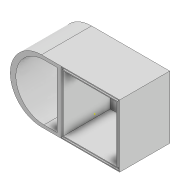
# Autodesk Inventor part: BetterPrototyp
Saved by Autodesk Inventor 2020 (Build 240168000, 168)
## iProperties
Created: 2021-06-29
Part Number: BetterPrototyp
Material: Generisch
Document SubType Name: Modeling
Designer: Julian Uhl
Density: 1 g/cm^3
Appearance: Vorgabe
Author: Julian Uhl
Autodesk Inventor part; units mm, degrees
ref_plane "YZ Plane" through (0, 0, 0) normal (1, 0, 0) x (0, 1, 0)
ref_plane "XZ Plane" through (0, 0, 0) normal (0, 1, 0) x (-1, 0, 0)
ref_plane "XY Plane" through (0, 0, 0) normal (0, 0, 1) x (1, 0, 0)
sketch "Skizze1" plane through (0, 0, 0) normal (0, 0, 1) x (1, 0, 0)
  line L0 (-160.1182, 0) -> (119.8818, 0) projected
  line L1 (0, -160.7697) -> (0, 119.2303) projected
  line L2 (-120.1182, 79.2303) -> (79.8818, 79.2303)
  line L3 (79.8818, 79.2303) -> (79.8818, -120.7697)
  line L4 (79.8818, -120.7697) -> (-120.1182, -120.7697)
  line L5 (-120.1182, -120.7697) -> (-120.1182, 79.2303)
  line L6 (-110.1182, 69.2303) -> (69.8818, 69.2303)
  line L7 (69.8818, 69.2303) -> (69.8818, -110.7697)
  line L8 (69.8818, -110.7697) -> (-110.1182, -110.7697)
  line L9 (-110.1182, -110.7697) -> (-110.1182, 69.2303)
  point P0 (0, 0)
  dimension "d0" = 200
  dimension "d1" = 200
  dimension "d2" = 10
  dimension "d3" = 10
  dimension "d4" = 10
  dimension "d5" = 10
  constraints: 16 end point, 4 parallel, 2 horizontal, 2 perpendicular
  measures "d0" distance between parallel lines of L4 L2
  measures "d1" distance between parallel lines of L5 L3
  measures "d2" distance between parallel lines of L2 L6
  measures "d3" distance between parallel lines of L5 L9
  measures "d4" distance between parallel lines of L3 L7
  measures "d5" distance between parallel lines of L4 L8
extrude "Extrusion1" add sketch "Skizze1" along normal blind 150 contours L5 L2 L1 L6 L9 L0 | L0 L9 L8 L1 L4 L5 | L1 L8 L7 L0 L3 L4 | L2 L3 L0 L7 L6 L1
sketch "Skizze2" plane through (-120.1182, -120.7697, 0) normal (-1, 0, 0) x (0, 0, 1)
  point P0 (0, 120.7697)
sketch "Skizze3" plane through (-120.1182, -120.7697, 0) normal (-1, 0, 0) x (0, 0, 1)
  point P0 (0, 120.7697)
sketch "Skizze4" plane through (-120.1182, -120.7697, 0) normal (-1, 0, 0) x (0, 0, 1)
  point P0 (0, 120.7697)
sketch "Skizze5" plane through (-120.1182, -120.7697, 0) normal (-1, 0, 0) x (0, 0, 1)
  point P0 (0, 120.7697)
sketch "Skizze6" plane through (-120.1182, -120.7697, 0) normal (-1, 0, 0) x (0, 0, 1)
  point P0 (0, 120.7697)
sketch "Skizze7" plane through (0, 0, 0) normal (0, 0, -1) x (-1, 0, 0)
  line L0 (120.1182, 79.2303) -> (120.1182, -120.7697) projected
  line L1 (120.1182, 79.2303) -> (170.1182, 79.2303)
  line L2 (170.1182, -120.7697) -> (120.1182, -120.7697)
  line L3 (120.1182, -120.7697) -> (120.1182, 79.2303)
  arc A0 (170.1182, -120.7697) -> (170.1182, 79.2303) centre (170.1182, -20.7697) ccw
  line L4 (120.1182, 69.2303) -> (162.1378, 69.2303)
  line L5 (162.1378, -110.7697) -> (120.1182, -110.7697)
  line L6 (120.1182, -110.7697) -> (120.1182, 69.2303)
  arc A1 (162.1378, -110.7697) -> (162.1378, 69.2303) centre (162.1378, -20.7697) ccw
  point P0 (0, 0)
  dimension "d9" = 10
  dimension "d10" = 10
  constraints: 12 end point, 4 point on circle, 4 tangent, 2 centre point, 2 horizontal, 2 parallel, 1 point on line
  measures "d9" distance between parallel lines of L1 L4
  measures "d10" distance between parallel lines of L2 L5
extrude "Extrusion2" add sketch "Skizze7" against normal blind 150 contours L1 A0 L2 L0 L5 A1 L4
sketch "Skizze8" plane through (-110.1182, -110.7697, 0) normal (1, 0, 0) x (0, 0, -1)
  line L0 (-150, 0) -> (-150, 180) projected
  line L1 (0, 0) -> (0, 180) projected
  line L2 (-150, 0) -> (0, 0)
  line L3 (0, 0) -> (0, 180)
  line L4 (0, 180) -> (-150, 180)
  line L5 (-150, 180) -> (-150, 0)
  point P0 (0, 110.7697)
  constraints: 8 end point, 2 parallel, 1 horizontal, 1 perpendicular
extrude "Extrusion3" add sketch "Skizze8" along normal blind 10
sketch "Skizze9" plane through (0, 0, 0) normal (0, 0, -1) x (-1, 0, 0)
  line L0 (-79.8818, 79.2303) -> (170.1182, 79.2303) projected
  line L1 (-79.8818, 79.2303) -> (120.1182, 79.2303)
  line L2 (120.1182, 79.2303) -> (120.1182, -110.7697)
  line L3 (120.1182, -110.7697) -> (-79.8818, -110.7697)
  line L4 (-79.8818, -110.7697) -> (-79.8818, 79.2303)
  arc A0 (170.1182, -120.7697) -> (170.1182, 79.2303) centre (170.1182, -20.7697) ccw projected
  arc A1 (170.1182, -120.7697) -> (170.1182, 79.2303) centre (170.1182, -20.7697) ccw
  line L5 (120.1182, 79.2303) -> (170.1182, 79.2303)
  line L6 (-79.8818, -120.7697) -> (170.1182, -120.7697) projected
  line L7 (120.1182, -120.7697) -> (170.1182, -120.7697)
  line L8 (120.1182, -110.7697) -> (-79.8818, -110.7697)
  line L9 (-79.8818, -110.7697) -> (-79.8818, -120.7697)
  line L10 (-79.8818, -120.7697) -> (120.1182, -120.7697)
  line L11 (120.1182, -120.7697) -> (120.1182, -110.7697)
  point P0 (0, 0)
  point P1 (-79.8818, -110.7697)
  constraints: 20 end point, 4 parallel, 2 collinear, 2 horizontal, 2 perpendicular, 2 point on circle, 1 centre point, 1 tangent
extrude "Extrusion4" add sketch "Skizze9" along normal blind 10
sketch "Skizze10" plane through (0, 0, 150) normal (0, 0, 1) x (1, 0, 0)
  point P0 (0, 0)
sketch "Skizze11" plane through (0, 0, 150) normal (0, 0, 1) x (1, 0, 0)
  line L0 (-107.6182, 76.7303) -> (77.3818, 76.7303)
  line L1 (77.3818, 76.7303) -> (77.3818, 71.09)
  line L2 (72.3818, 71.7303) -> (-102.6182, 71.7303)
  line L3 (-107.6182, 71.09) -> (-107.6182, 76.7303)
  line L4 (77.3818, -113.2626) -> (77.3818, -118.2697)
  line L5 (77.3818, -118.2697) -> (-107.6182, -118.2697)
  line L6 (-107.6182, -118.2697) -> (-107.6182, -113.2626)
  line L7 (77.3818, -113.2626) -> (77.3818, 71.09)
  line L8 (72.3818, 71.7303) -> (72.3818, -113.2697)
  line L9 (-102.6182, 71.7303) -> (-102.6182, -113.2697)
  line L10 (-107.6182, -113.2626) -> (-107.6182, 71.09)
  line L11 (-107.6182, -113.2626) -> (-107.6182, -113.2626)
  line L12 (-102.6182, -113.2697) -> (72.3818, -113.2697)
  line L13 (77.3818, -113.2626) -> (77.3818, -113.2626)
  line L14 (79.8818, 79.2303) -> (-170.1182, 79.2303) projected
  line L15 (79.8818, -120.7697) -> (79.8818, 79.2303) projected
  line L16 (-100.1182, 69.2303) -> (69.8818, 69.2303) projected
  line L17 (69.8818, 69.2303) -> (69.8818, -110.7697) projected
  line L18 (69.8818, -110.7697) -> (-100.1182, -110.7697) projected
  line L19 (-170.1182, -120.7697) -> (79.8818, -120.7697) projected
  line L20 (-100.1182, 69.2303) -> (-100.1182, -110.7697) projected
  point P0 (0, 0)
  dimension "d17" = 2.5
  dimension "d18" = 2.5
  dimension "d19" = 2.5
  dimension "d20" = 2.5
  dimension "d21" = 2.5
  dimension "d22" = 2.5
  dimension "d23" = 2.5
  dimension "d24" = 2.5
  dimension "d25" = 5
  dimension "d26" = 5
  constraints: 28 end point, 8 parallel, 4 horizontal, 4 perpendicular
  measures "d17" distance between parallel lines of L14 L0
  measures "d18" distance between parallel lines of L15 L7
  measures "d19" distance between parallel lines of L16 L2
  measures "d20" distance between parallel lines of L17 L8
  measures "d21" distance between parallel lines of L15 L4
  measures "d22" distance between parallel lines of L12 L18
  measures "d23" distance between parallel lines of L19 L5
  measures "d24" distance between parallel lines of L20 L9
  measures "d25" distance between parallel lines of L9 L6
  measures "d26" distance between parallel lines of L9 L10
extrude "Extrusion5" cut sketch "Skizze11" against normal blind 5 contours L0 L1 L7 L4 L5 L6 L10 L3
sketch "Skizze12" plane through (0, 0, 0) normal (0, 0, 1) x (1, 0, 0)
  line L0 (-100.1182, 69.2303) -> (69.8818, 69.2303) projected
  line L1 (69.8818, 69.2303) -> (69.8818, -110.7697) projected
  line L2 (-20.1182, -15.7697) -> (-10.1182, -15.7697)
  line L3 (-10.1182, -15.7697) -> (-10.1182, -25.7697)
  line L4 (-10.1182, -25.7697) -> (-20.1182, -25.7697)
  line L5 (-20.1182, -25.7697) -> (-20.1182, -15.7697)
  point P0 (0, 0)
  point P1 (-15.1182, -20.7697)
  dimension "d29" = 90
  dimension "d30" = 85
  dimension "d31" = 5
  dimension "d32" = 5
  dimension "d33" = 5
  dimension "d34" = 5
  constraints: 8 end point, 2 parallel, 1 horizontal, 1 perpendicular
  measures "d29" distance from line of L0 point (-15.118, -20.77)
  measures "d30" distance from line of L1 point (-15.118, -20.77)
  measures "d31" distance from line of L2 point (-15.118, -20.77)
  measures "d32" distance from line of point (-15.118, -20.77) L4
  measures "d33" distance from line of point (-15.118, -20.77) L5
  measures "d34" horizontal distance of L2.end point (-15.118, -20.77)
extrude "Extrusion6" cut sketch "Skizze12" against normal blind 5
